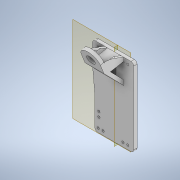
# Autodesk Inventor part: Fastener
Saved by Autodesk Inventor 2022 (Build 260153000, 153)
## iProperties
Created: 2023-10-19
Part Number: Fastener
Material: Типовые
Document SubType Name: Modeling
Designer: user
Density: 1 g/cm^3
Appearance: По умолчанию
Author: user
## iProperties of the stored document Fastener horizontal 3_3DПЕЧАТЬ.ipt
Created: 2023-10-22
Part Number: Fastener horizontal 3_3DПЕЧАТЬ
Material: Типовые
Document SubType Name: Modeling
Designer: user
Density: 1 g/cm^3
Appearance: По умолчанию
Author: user
Autodesk Inventor part; units mm, degrees
ref_plane "YZ Plane" through (0, 0, 0) normal (1, 0, 0) x (0, 1, 0)
ref_plane "XZ Plane" through (0, 0, 0) normal (0, 1, 0) x (-1, 0, 0)
ref_plane "XY Plane" through (0, 0, 0) normal (0, 0, 1) x (1, 0, 0)
ref_plane "РабПлоскость1" through (0, 0, 0) normal (0, 0, 1) x (1, 0, 0)
sketch "Эскиз1" plane through (0, 0, 0) normal (0, 0, 1) x (1, 0, 0)
  line L0 (15.9535, 22.685) -> (15.9535, 17.285) projected
  line L1 (15.9535, 17.285) -> (5.5535, 17.285) projected
  line L2 (5.5535, 17.285) -> (5.5535, 22.685) projected
  line L3 (5.5535, 22.685) -> (15.9535, 22.685) projected
  line L4 (15.9535, -17.315) -> (15.9535, -22.715) projected
  line L5 (15.9535, -22.715) -> (5.5535, -22.715) projected
  line L6 (5.5535, -22.715) -> (5.5535, -17.315) projected
  line L7 (5.5535, -17.315) -> (15.9535, -17.315) projected
  arc A0 (-2.3465, 28.685) -> (-4.3465, 26.685) centre (-2.3465, 26.685) ccw projected
  line L8 (-4.3465, 12.1) -> (-4.3465, 26.685) projected
  arc A1 (-5.6809, 10.2141) -> (-4.3465, 12.1) centre (-6.3465, 12.1) ccw projected
  line L9 (-11.5122, 8.156) -> (-5.6809, 10.2141) projected
  arc A2 (-11.5122, 8.156) -> (-12.8465, 6.27) centre (-10.8465, 6.27) ccw projected
  line L10 (-12.8465, -1.915) -> (-12.8465, 6.27) projected
  arc A3 (-12.8465, -1.915) -> (-10.8465, -3.915) centre (-10.8465, -1.915) ccw projected
  line L11 (-4.6465, -3.915) -> (-10.8465, -3.915) projected
  arc A4 (-2.6465, -5.915) -> (-4.6465, -3.915) centre (-4.6465, -5.915) ccw projected
  line L12 (-2.6465, -26.715) -> (-2.6465, -5.915) projected
  arc A5 (-2.6465, -26.715) -> (-0.6465, -28.715) centre (-0.6465, -26.715) ccw projected
  line L13 (23.8535, -28.715) -> (-0.6465, -28.715) projected
  arc A6 (23.8535, -28.715) -> (25.8535, -26.715) centre (23.8535, -26.715) ccw projected
  line L14 (25.8535, 26.685) -> (25.8535, -26.715) projected
  arc A7 (25.8535, 26.685) -> (23.8535, 28.685) centre (23.8535, 26.685) ccw projected
  line L15 (-2.3465, 28.685) -> (23.8535, 28.685) projected
  circle A8 centre (18.0535, 25.685) radius 0.8 projected
  circle A9 centre (21.6535, 25.685) radius 0.8 projected
  circle A10 centre (21.6535, -25.715) radius 0.8 projected
  circle A11 centre (18.0535, -25.715) radius 0.8 projected
  circle A12 centre (0.3535, -18.515) radius 0.8 projected
  circle A13 centre (0.3535, -14.915) radius 0.8 projected
  circle A14 centre (-1.3465, 16.885) radius 0.8 projected
  circle A15 centre (-1.3465, 20.485) radius 0.8 projected
  circle A16 centre (-0.1465, 25.685) radius 0.8 projected
  circle A17 centre (3.4535, 25.685) radius 0.8 projected
  circle A18 centre (-0.1465, -25.715) radius 0.8 projected
  circle A19 centre (3.4535, -25.715) radius 0.8 projected
  line L16 (-4.3465, 12.1) -> (-2.6465, -5.915)
  circle A20 centre (51.6035, 35.685) radius 3
  circle A21 centre (51.6035, 35.685) radius 6
  line L17 (11.6035, -28.715) -> (11.6035, 28.685) construction
  line L18 (56.9244, 32.9123) -> (25.8535, -26.715)
  line L19 (50.1799, 41.5137) -> (-2.3465, 28.685)
  point P0 (0, 0)
  point P1 (-2.6818, -5.5409)
  dimension "d11" = 6
  dimension "d12" = 12
  dimension "d13" = 7
  dimension "d14" = 40
  constraints: 8 end point, 2 centre point, 2 point on circle, 2 tangent, 1 coincident, 1 midpoint, 1 perpendicular, 1 point on line
  measures "d11" diameter of A20
  measures "d12" diameter of A21
  measures "d13" distance from line of L15 A20.centre
  measures "d14" distance from line of A20.centre L17
extrude "Выдавливание1" add sketch "Эскиз1" along normal blind 2.5 contours L0 L1 L2 L3 | L4 L5 L6 L7 | L15 A7 L14 A6 L13 A5 L12 A4 L16 L8 A0
ref_plane "РабПлоскость3" through (11.6035, -26.715, 0) normal (-1, 0, 0) x (0, 0, 1)
sketch "Эскиз7" plane through (11.6035, -26.715, 0) normal (-1, 0, 0) x (0, 0, 1)
  line L0 (14.7, 53.1663) -> (19.831, 66.1921)
  line L1 (19.831, 66.1921) -> (22.1571, 65.2759)
  line L2 (22.1571, 65.2759) -> (17.026, 52.25)
  line L3 (17.026, 52.25) -> (14.7, 53.1663)
  line L4 (17.026, 52.25) -> (2.5, 37.3616)
  line L5 (2.5, 38.815) -> (2.5, 21.1741) projected
  line L6 (14.7, 53.1663) -> (2.5, 55.4)
  line L7 (12.3647, 51.0523) -> (2.5, 40.9415)
  line L8 (2.5, 0) -> (2.5, 53.4) projected
  line L9 (12.3647, 51.0523) -> (2.5, 52.8584)
  line L10 (2.5, 53.4) -> (2.5, 55.4) projected
  line L11 (18.0515, 61.6744) -> (2.5, 55.4)
  point P0 (0, 26.715)
  dimension "d48" = 14
  dimension "d49" = 2.5
  dimension "d50" = 2.5
  dimension "d51" = 21.5
  dimension "d52" = 12.2
  dimension "d53" = 2.5
  constraints: 18 end point, 4 parallel, 4 point on line, 1 perpendicular
  measures "d48" distance of L1.end L2.end
  measures "d49" distance of L0.end L1.end
  measures "d50" distance between parallel lines of L4 L7
  measures "d51" angle of L8 L0
  measures "d52" distance from line of L8 L0.start
  measures "d53" distance between parallel lines of L9 L6
extrude "Выдавливание5" add sketch "Эскиз7" along normal mid plane 2.5 contours L9 L7 L8
extrude "Выдавливание6" add sketch "Эскиз7" along normal mid plane 14 contours L0 L1 L2 L3 | L3 L4 L5 L8 L7 L9 L10 L6
fillet "Сопряжение3" radius 7 2 edges at (18.6035, 39.019, 20.994) (4.6035, 39.019, 20.994)
extrude "Выдавливание7" add sketch "Эскиз7" along normal blind 2 from surface at -7 contours L6 L11 L0
extrude "Выдавливание8" add sketch "Эскиз7" against normal blind 2 from surface at 7 contours L6 L11 L0
sketch "Эскиз8" plane through (4.6035, 25.535, 17.026) normal (0, -0.3665012, 0.9304176) x (1, 0, 0)
  circle A0 centre (7, 7) radius 3
  arc A1 (14, 7) -> (0, 7) centre (7, 7) ccw projected
  line L0 (14, 7) -> (14, 9.1445) projected
  line L1 (14, 7) -> (14, 14)
  line L2 (14, 14) -> (7, 14)
  arc A2 (13.6634, 9.1445) -> (0.3366, 9.1445) centre (7, 7) ccw projected
  line L3 (7, 14) -> (0, 14)
  arc A3 (0.3366, 9.1445) -> (0, 7) centre (7, 7) ccw projected
  line L4 (0, 14) -> (0, 7)
  circle A4 centre (7, 7) radius 7
  point P0 (-4.6035, -29.9983)
  point P1 (0, 7)
  point P2 (14, 7)
  dimension "d63" = 6
  constraints: 8 end point, 2 centre point, 2 concentric, 2 point on circle, 2 tangent, 1 coincident, 1 perpendicular, 1 point on line, 1 vertical
  measures "d63" diameter of A0
extrude "Выдавливание9" cut sketch "Эскиз8" against normal blind 10 contours A0 | A1 L2 L1 L0 | L4 L3 A1
extrude "Выдавливание10" cut sketch "Эскиз8" against normal blind 10 from surface at -2.5 contours A4 A1
fillet "Сопряжение4" radius 2 2 edges at (5.1227, 32.3544, 11.5947) (18.0842, 32.3544, 11.5947)
